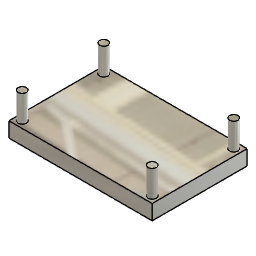
ecra+Pi+Pico (Autodesk Fusion 360 design; units mm, degrees)
Autodesk Fusion 360 part; units mm, degrees
sketch "Sketch1" plane through (0, 0, 0) normal (0, 1, 0) x (1, 0, 0)
  line L0 (43, -28.5) -> (-43, -28.5)
  line L1 (-43, -28.5) -> (-43, 28.5)
  line L2 (-43, 28.5) -> (43, 28.5)
  line L3 (43, 28.5) -> (43, -28.5)
  line L4 (43, -28.5) -> (-43, 28.5) construction
  line L5 (-43, -28.5) -> (43, 28.5) construction
  line L6 (43, -28.5) -> (39, -28.5)
  line L7 (39, -28.5) -> (39, -24.5)
  line L8 (39, -24.5) -> (43, -24.5)
  line L9 (43, -24.5) -> (43, -28.5)
  circle A0 centre (39, -24.5) radius 2.5
  line L10 (52.3114, 0) -> (-55.6196, 0)
  line L11 (0, 36.5366) -> (0, -32.8551)
  circle A1 centre (-39, -24.5) radius 2.5
  circle A2 centre (39, 24.5) radius 2.5
  circle A3 centre (-39, 24.5) radius 2.5
  dimension "d1" = 86
  dimension "d2" = 57
  dimension "d5" = 4
  dimension "d6" = 4
  dimension "d7" = 5
  constraint horizontal L0
  constraint perpendicular L0 L1
  constraint parallel L0 L2
  constraint parallel L1 L3
  constraint coincident L4 origin
  constraint coincident L5 origin
  constraint horizontal L6
  constraint vertical L7
  constraint horizontal L8
  constraint vertical L9
  constraint coincident L7.end L8.start
  constraint perpendicular L3 L10
  constraint vertical L11
  constraint symmetric A0 L11 A1
  constraint symmetric A0 L10 A2
  constraint symmetric L10 A1 A3
  measures "d1" distance of L1.end L2.end
  measures "d2" distance of L0.end L1.end
  measures "d5" distance of L0.start L6.end
  measures "d6" distance of L0.start L8.end
  measures "d7" diameter of A0
extrude "Extrude1" add sketch "Sketch1" along normal blind 9 contours L0 L3 L6 L7 L8 L9 A0 | L0 L3 L7 L8 A0 L10 L11 | L0 L1 L10 L11 | L7 L8 A0 | L7 L8 A0 | L2 L3 L10 L11 | L1 L2 L10 L11 | A1 | A2 | A3
extrude "Extrude2" add sketch "Sketch1" along normal blind 25 contours L7 L8 A0 | L7 L8 A0 | A1 | A2 | A3
